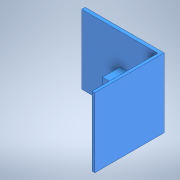
# Autodesk Inventor part: Pieza2
Saved by Autodesk Inventor 2021 (Build 250183000, 183)
## iProperties
Created: 2022-08-16
Part Number: Pieza2
Material: Genérico
Document SubType Name: Modeling
Designer: arthu
Density: 1 g/cm^3
Appearance: Cian
Author: arthu
Autodesk Inventor part; units mm, degrees
ref_plane "YZ Plane" through (0, 0, 0) normal (1, 0, 0) x (0, 1, 0)
ref_plane "XZ Plane" through (0, 0, 0) normal (0, 1, 0) x (-1, 0, 0)
ref_plane "XY Plane" through (0, 0, 0) normal (0, 0, 1) x (1, 0, 0)
sketch "Boceto1" plane through (0, 0, 0) normal (0, 0, 1) x (1, 0, 0)
  line L0 (175, -125) -> (-175, -125)
  line L1 (-175, -125) -> (-175, 125)
  line L2 (-175, 125) -> (175, 125)
  line L3 (175, 125) -> (175, -125)
  line L4 (175, -125) -> (-175, 125) construction
  line L5 (-175, -125) -> (175, 125) construction
  line L6 (-175, 125) -> (-165, 125) construction
  line L7 (-175, 125) -> (-275, 125)
  line L8 (-275, 125) -> (-275, 185)
  line L9 (-275, 185) -> (-175, 185)
  line L10 (-175, 185) -> (-175, 125)
  line L11 (-275, 185) -> (275, 185)
  line L12 (275, 185) -> (275, -365)
  line L13 (275, -365) -> (-275, -365)
  line L14 (-275, -365) -> (-275, 185)
  point P0 (0, 0)
  dimension "d0" = 350
  dimension "d1" = 250
  dimension "d4" = 100
  dimension "d5" = 60
  dimension "d6" = 550
  dimension "d7" = 550
  constraints: 30 end point, 6 parallel, 4 horizontal, 3 perpendicular, 2 midpoint
  measures "d0" distance of L1.end L2.end
  measures "d1" distance of L0.end L1.end
  measures "d4" distance of L8.end L9.end
  measures "d5" distance of L7.end L8.end
  measures "d6" distance of L12.end L13.end
  measures "d7" distance of L11.end L12.end
extrude "Extrusión1" add sketch "Boceto1" along normal blind 300
extrude "Extrusión2" add sketch "Boceto1" along normal blind 49 contours L0 L1 L2 L3
sketch "Boceto2" plane through (-275, -365, 0) normal (-1, 0, 0) x (0, 0, 1)
  line L0 (0, 550) -> (0, 0) projected
  line L1 (0, 0) -> (50, 0)
  line L2 (50, 0) -> (50, 1000)
  line L3 (50, 1000) -> (0, 1000)
  line L4 (0, 1000) -> (0, 0)
  point P0 (0, 365)
  dimension "d12" = 50
  dimension "d13" = 1000
  constraints: 8 end point, 2 parallel, 1 horizontal, 1 perpendicular
  measures "d12" distance of L3.end L2.end
  measures "d13" distance of L2.end L1.end
extrude "Extrusión3" add sketch "Boceto2" along normal mid plane 1100
sketch "Boceto3" plane through (275, -365, 300) normal (1, 0, 0) x (0, 0, -1)
  line L0 (300, 0) -> (300, 1000) projected
  line L1 (300, 0) -> (-700, 0)
  line L2 (-700, 0) -> (-700, 1000)
  line L3 (-700, 1000) -> (300, 1000)
  line L4 (300, 1000) -> (300, 0)
  point P0 (300, 365)
  dimension "d16" = 1000
  constraints: 8 end point, 2 parallel, 1 horizontal, 1 perpendicular
  measures "d16" distance of L2.end L3.end
extrude "Extrusión4" add sketch "Boceto3" along normal blind 40
